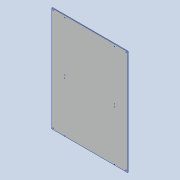
# Autodesk Inventor part: 0008-10-017 Heated bed
Saved by Autodesk Inventor 2020 (Build 240168000, 168)
## iProperties
Created: 2021-02-27
Part Number: 0008-10-017 Heated bed
Material: Aluminum 6061
Document SubType Name: Modeling
Designer: Iulian Bors
Density: 2.7 g/cm^3
Appearance: Aluminum - Flat
Mass: 1129.02 g
Surface Area: 2836.81 cm^2
Volume: 418.157 cm^3
Description: Pat incalzit
Author: Iulian Bors
Subject: 017
Autodesk Inventor part; units mm, degrees
ref_plane "YZ Plane" through (0, 0, 0) normal (1, 0, 0) x (0, 1, 0)
ref_plane "XZ Plane" through (0, 0, 0) normal (0, 1, 0) x (-1, 0, 0)
ref_plane "XY Plane" through (0, 0, 0) normal (0, 0, 1) x (1, 0, 0)
sketch "Sketch1" plane through (0, 0, 0) normal (0, 0, 1) x (1, 0, 0)
  line L0 (-158.5, 220) -> (158.5, 220)
  line L1 (158.5, 220) -> (158.5, -220)
  line L2 (158.5, -220) -> (-158.5, -220)
  line L3 (-158.5, -220) -> (-158.5, 220)
  line L4 (-153.5, 215) -> (153.5, 215) construction
  line L5 (153.5, 215) -> (153.5, -215) construction
  line L6 (153.5, -215) -> (-153.5, -215) construction
  line L7 (-153.5, -215) -> (-153.5, 215) construction
  circle A0 centre (-153.5, 215) radius 2
  circle A1 centre (153.5, 215) radius 2
  circle A2 centre (153.5, -215) radius 2
  circle A3 centre (-153.5, -215) radius 2
  point P0 (0, 0)
  point P1 (0, 220)
  point P2 (-158.5, 0)
  point P3 (0, 215)
  point P4 (-153.5, 0)
  dimension "d0" = 440
  dimension "d1" = 317
  dimension "d3" = 5
  dimension "d4" = 5
  dimension "d5" = 4
  constraints: 16 end point, 4 centre point, 4 coincident, 4 midpoint, 4 parallel, 3 equal radius, 2 horizontal, 2 horizontal alignment, 2 perpendicular, 2 vertical alignment
  measures "d0" distance of L2.end L0.start
  measures "d1" distance of L1.end L2.end
  measures "d3" distance between parallel lines of L3 L7
  measures "d4" distance between parallel lines of L0 L4
  measures "d5" diameter of A0
extrude "Extrusion1" add sketch "Sketch1" along normal blind 3
sketch "Sketch2" plane through (0, 0, 0) normal (0, 0, -1) x (-1, 0, 0)
  circle A0 centre (0, 0) radius 1.5
  dimension "d8" = 3
  constraints: 1 centre point, 1 coincident
  measures "d8" diameter of A0
extrude "Extrusion2" cut sketch "Sketch2" against normal blind 2
sketch "Sketch3" plane through (0, 0, 0) normal (0, 0, -1) x (-1, 0, 0)
  circle A0 centre (104.5, 211.5) radius 1.5 projected
  circle A1 centre (104.5, 2.5) radius 1.5 projected
  circle A2 centre (-104.5, 2.5) radius 1.5 projected
  circle A3 centre (-104.5, 211.5) radius 1.5 projected
  circle A4 centre (-104.5, -8.5) radius 1.5 projected
  circle A5 centre (-104.5, -217.5) radius 1.5 projected
  circle A6 centre (104.5, -217.5) radius 1.5 projected
  circle A7 centre (104.5, -8.5) radius 1.5 projected
  point P0 (0, 0)
  point P1 (-1.0607, -1.0607)
hole "Hole1" at (-104.5, 211.5, 0) at (-104.5, 2.5, 0) at (-104.5, -8.5, 0) at (104.5, -8.5, 0) at (104.5, 2.5, 0) at (104.5, 211.5, 0) at (-104.5, -217.5, 0) at (104.5, -217.5, 0) direction (0, 0, 1) diameter 2.5 end through all
body "Solid1"
